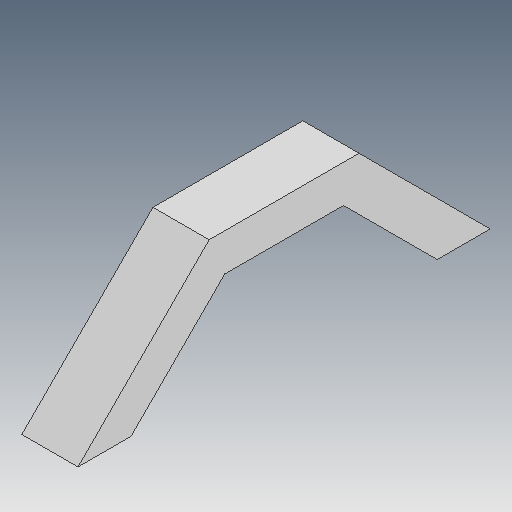
# Autodesk Inventor part: Handle
Saved by Autodesk Inventor 2027 (Build 310192060, 192F)
## iProperties
Created: 2026-07-28
Part Number: Handle
Material: Generic
Document SubType Name: Modeling
Designer: prest
Density: 1 g/cm^3
Appearance: Default
Author: prest
Autodesk Inventor part; units mm, degrees
ref_plane "YZ Plane" through (0, 0, 0) normal (1, 0, 0) x (0, 1, 0)
ref_plane "XZ Plane" through (0, 0, 0) normal (0, 1, 0) x (-1, 0, 0)
ref_plane "XY Plane" through (0, 0, 0) normal (0, 0, 1) x (1, 0, 0)
sketch "Sketch1" plane through (0, 0, 0) normal (1, 0, 0) x (0, 1, 0)
  line L0 (0, 110) -> (70, 40)
  line L1 (70, 40) -> (70, -40)
  line L2 (70, -40) -> (0, -110)
  line L3 (0, 110) -> (0, -110) construction
  line L4 (0, -81.7157) -> (50, -31.7157)
  line L5 (50, -31.7157) -> (50, 31.7157)
  line L6 (50, 31.7157) -> (0, 81.7157)
  line L7 (0, -110) -> (0, -81.7157)
  line L8 (0, 81.7157) -> (0, 110)
  point P0 (0, 0)
  point P1 (70, 0)
  point P2 (0, 0)
  point P3 (50, 0)
  dimension "d0" = 220
  dimension "d2" = 45
  dimension "d3" = 20
  dimension "d4" = 50
  dimension "d5" = 20
  constraints: 18 end point, 3 midpoint, 2 collinear, 2 horizontal alignment, 2 perpendicular, 2 point on line, 2 vertical, 2 vertical alignment
  measures "d0" distance of L2.end L0.start
  measures "d2" angle of L3 L0
  measures "d3" distance between parallel lines of L0 L6
  measures "d4" distance from line of point (0, 0) L5
  measures "d5" distance between parallel lines of L1 L5
extrude "Extrusion1" add sketch "Sketch1" along normal mid plane 30
body "Solid1"
